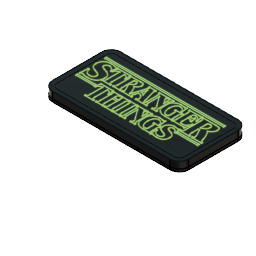
Stranger Things Lightbox (Autodesk Fusion 360 design; units mm, degrees)
part number: 2026-01-11-10-43-36-341
part number: 2026-01-17-18-05-47-932
part number: 2026-01-17-18-06-36-939
part number: 2026-01-17-18-06-53-033
Autodesk Fusion 360 part; units mm, degrees
sketch "Sketch1" plane through (0, 0, 0) normal (0, 0, 1) x (1, 0, 0)
  line L0 (-110, 55) -> (110, 55)
  line L1 (110, 55) -> (110, -55)
  line L2 (110, -55) -> (-110, -55)
  line L3 (-110, -55) -> (-110, 55)
  line L4 (-110, 55) -> (110, -55) construction
  line L5 (110, 55) -> (-110, -55) construction
  dimension "d1" = 220
  dimension "d2" = 110
  constraint horizontal L0
  constraint perpendicular L0 L1
  constraint parallel L0 L2
  constraint parallel L1 L3
  constraint coincident L4 origin
  constraint coincident L5 origin
  measures "d1" distance of L1.end L2.end
  measures "d2" distance of L0.end L1.end
extrude "Extrude1" add sketch "Sketch1" along normal blind 11 makes body 1
fillet "Fillet1" radius 15 4 edges at (110, 55, 5.5) (110, -55, 5.5) (-110, -55, 5.5) (-110, 55, 5.5) on bodies 1
shell "Shell1" thickness 7 removed faces 1 at (-31.6667, -18.3333, 0) on bodies 1
ref_plane "WorkPlane1" through (0, 0, 0) normal (0, 0, -1) x (-1, 0, 0)
sketch "Sketch4" plane through (0, 0, 0) normal (0, 0, 1) x (1, 0, 0)
  line L0 (-95, 55) -> (95, 55) construction
  line L1 (95, 48) -> (-95, 48) construction
  line L2 (0, 55) -> (0, 48) construction
  line L3 (95, 55) -> (95, 48) construction
  line L4 (0, 51.5) -> (95, 51.5) construction
  circle A0 centre (85, 51.5) radius 2.55
  line L5 (20, 0) -> (2.5, 0) construction
  circle A1 centre (85, -51.5) radius 2.55
  line L6 (0, 2.5) -> (0, 20) construction
  circle A2 centre (-85, 51.5) radius 2.55
  circle A3 centre (-85, -51.5) radius 2.55
  circle A4 centre (0, 51.5) radius 2.55
  line L7 (-103, 0) -> (-110, 0) construction
  circle A5 centre (-106.5, 0) radius 2.55
  circle A6 centre (0, -51.5) radius 2.55
  circle A7 centre (106.5, 0) radius 2.55
  point P0 (85, 51.5)
  dimension "d13" = 10
  dimension "d14" = 5.1
  dimension "d87" = 5.1
  dimension "d88" = 5.1
  constraint midpoint L0 L2.start
  constraint midpoint L1 L2.end
  constraint coincident L0.end L3.start
  constraint coincident L1.start L3.end
  constraint midpoint L2 L4.start
  constraint midpoint L3 L4.end
  constraint coincident L4 P0
  constraint coincident P0 A0.centre
  constraint symmetric A0 L5 A1
  constraint symmetric A0 L6 A2
  constraint symmetric A1 L6 A3
  constraint coincident L4.start A4.centre
  constraint horizontal L7
  constraint midpoint L7 A5.centre
  constraint symmetric L5 A4 A6
  constraint symmetric L6 A5 A7
  measures "d13" distance of L4.end P0
  measures "d14" diameter of A0
  measures "d87" diameter of A4
  measures "d88" diameter of A5
move_face "OffsetFaces1" offset -6 1 faces at (-31.6667, -16, 4) on bodies 1
extrude "Extrude4" cut sketch "Sketch4" along normal blind 3 bodies 1
sketch "Sketch5" plane through (0, 0, 0) normal (0, 0, -1) x (-1, 0, 0)
  line L0 (110, -55) -> (-110, -55)
  line L1 (-110, -55) -> (-110, 55)
  line L2 (-110, 55) -> (110, 55)
  line L3 (110, 55) -> (110, -55)
  line L4 (110, -55) -> (-110, 55) construction
  line L5 (-110, -55) -> (110, 55) construction
  dimension "d20" = 220
  dimension "d21" = 110
  constraint horizontal L0
  constraint perpendicular L0 L1
  constraint parallel L0 L2
  constraint parallel L1 L3
  constraint coincident L4 origin
  constraint coincident L5 origin
  measures "d20" distance of L1.end L2.end
  measures "d21" distance of L0.end L1.end
extrude "Extrude6" add sketch "Sketch5" along normal blind 4 separate body makes body 2
fillet "Fillet2" radius 15 4 edges at (110, 55, -2) (110, -55, -2) (-110, -55, -2) (-110, 55, -2) on bodies 2
extrude "Extrude7" cut sketch "Sketch4" against normal blind 3 bodies 2
sketch "Sketch6" plane through (0, 0, -4) normal (0, 0, -1) x (1, 0, 0)
  arc A0 (-110, -40) -> (-95, -55) centre (-95, -40) ccw
  line L0 (-95, -55) -> (95, -55)
  arc A1 (95, -55) -> (110, -40) centre (95, -40) ccw
  line L1 (110, -40) -> (110, 40)
  arc A2 (110, 40) -> (95, 55) centre (95, 40) ccw
  line L2 (95, 55) -> (-95, 55)
  arc A3 (-95, 55) -> (-110, 40) centre (-95, 40) ccw
  line L3 (-110, 40) -> (-110, -40)
  circle A4 centre (0, 40) radius 4.25
  dimension "d28" = 15
  dimension "d53" = 8.5
  measures "d28" distance of L2 A4.centre
  measures "d53" diameter of A4
sketch "Sketch7" plane through (0, 0, -4) normal (0, 0, -1) x (1, 0, 0)
  arc A0 (-110, -40) -> (-95, -55) centre (-95, -40) ccw
  line L0 (-95, -55) -> (95, -55)
  arc A1 (95, -55) -> (110, -40) centre (95, -40) ccw
  line L1 (110, -40) -> (110, 40)
  arc A2 (110, 40) -> (95, 55) centre (95, 40) ccw
  line L2 (95, 55) -> (-95, 55)
  arc A3 (-95, 55) -> (-110, 40) centre (-95, 40) ccw
  line L3 (-110, 40) -> (-110, -40)
  line L4 (0, 55) -> (95, 55) construction
  line L5 (47.5, 55) -> (57.5, 55)
  line L6 (57.5, 55) -> (57.5, 30.0008)
  line L7 (57.5, 30.0008) -> (37.5, 30.0008)
  line L8 (37.5, 30.0008) -> (37.8912, 55)
  line L9 (0, -2.5) -> (0, -20)
  line L10 (-57.5, 30.0008) -> (-37.5, 30.0008)
  line L11 (-57.5, 55) -> (-57.5, 30.0008)
  line L12 (-37.5, 30.0008) -> (-37.8912, 55)
  point P0 (47.5, 55)
  dimension "d31" = 10
  dimension "d32" = 20
  constraint midpoint L2 L4.start
  constraint coincident A2.end L2.start
  constraint midpoint L4 P0
  constraint coincident P0 L5.start
  constraint parallel L2 L5
  constraint perpendicular L5 L6
  constraint perpendicular L6 L7
  constraint coincident L2 L8.end
  constraint symmetric L5.end L9 L11.start
  constraint symmetric L6.end L9 L10.start
  constraint symmetric L7.end L9 L10.end
  constraint symmetric L8.end L9 L12.end
  measures "d31" distance of P0 L5.end
  measures "d32" distance of L6.end L7.end
extrude "Extrude9" add sketch "Sketch7" along normal blind 20 separate body contours L2 L10 L11 L12 | L2 L5 L6 L7 L8 makes body 3 at (-37.6304, -38.3339, -10.6667) makes body 4 at (37.6304, -38.3339, -17.3333)
sketch "Sketch8" plane through (57.5, 0, 0) normal (1, 0, 0) x (0, 1, 0)
  line L0 (-55, -4) -> (-55, -24)
  line L1 (-55, -24) -> (-30.0008, -24)
  line L2 (-30.0008, -24) -> (-30.0008, -4)
  circle A0 centre (-30.0008, -24) radius 18.75
  line L3 (-30.0008, -4) -> (-55, -4)
  dimension "d35" = 37.5
  constraint coincident L1.end L2.start
  measures "d35" diameter of A0
extrude "Extrude10" cut sketch "Sketch8" against normal blind 120 contours L1 L2 A0 picked at (-42.4372, -23.1105) bodies 4 2 3
fillet "Fillet3" radius 10 4 edges at (-47.5, -30.0008, -5.25) (-47.6467, -48.7508, -24) (47.6467, -48.7508, -24) (47.5, -30.0008, -5.25) on bodies 3 4
sketch "Sketch9" plane through (0, 0, 0) normal (0, 0, 1) x (-1, 0, 0)
  arc A0 (95, -55) -> (110, -40) centre (95, -40) ccw
  line L0 (110, -40) -> (110, 40)
  arc A1 (110, 40) -> (95, 55) centre (95, 40) ccw
  line L1 (95, 55) -> (-95, 55)
  arc A2 (-95, 55) -> (-110, 40) centre (-95, 40) ccw
  line L2 (-110, 40) -> (-110, -40)
  arc A3 (-110, -40) -> (-95, -55) centre (-95, -40) ccw
  line L3 (-95, -55) -> (95, -55)
  circle A4 centre (-85, -51.5) radius 2.55
  circle A5 centre (85, -51.5) radius 2.55
  circle A6 centre (-85, 51.5) radius 2.55
  circle A7 centre (85, 51.5) radius 2.55
  line L4 (102.8, -40) -> (102.8, 40)
  arc A8 (102.8, 40) -> (95, 47.8) centre (95, 40) ccw
  line L5 (95, 47.8) -> (-95, 47.8)
  arc A9 (-95, 47.8) -> (-102.8, 40) centre (-95, 40) ccw
  line L6 (-102.8, 40) -> (-102.8, -40)
  arc A10 (-102.8, -40) -> (-95, -47.8) centre (-95, -40) ccw
  line L7 (-95, -47.8) -> (95, -47.8)
  arc A11 (95, -47.8) -> (102.8, -40) centre (95, -40) ccw
  line L8 (101.6, -40) -> (101.6, 40)
  arc A12 (101.6, 40) -> (95, 46.6) centre (95, 40) ccw
  line L9 (95, 46.6) -> (-95, 46.6)
  arc A13 (-95, 46.6) -> (-101.6, 40) centre (-95, 40) ccw
  line L10 (-101.6, 40) -> (-101.6, -40)
  arc A14 (-101.6, -40) -> (-95, -46.6) centre (-95, -40) ccw
  line L11 (-95, -46.6) -> (95, -46.6)
  arc A15 (95, -46.6) -> (101.6, -40) centre (95, -40) ccw
  circle A16 centre (-106.5, 0) radius 2.55
  circle A17 centre (0, 51.5) radius 2.55
  circle A18 centre (106.5, 0) radius 2.55
  circle A19 centre (0, -51.5) radius 2.55
  dimension "d40" = -7.2
  dimension "d45" = -1.2
extrude "Extrude11" cut sketch "Sketch9" against normal blind 4 contours L4 A8 L5 A9 L6 A10 L7 A11 | L8 A12 L9 A13 L10 A14 L11 A15 bodies 3 4 2
extrude "Extrude12" add sketch "Sketch9" against normal blind 4 separate body contours L4 A8 L5 A9 L6 A10 L7 A11 | L8 A12 L9 A13 L10 A14 L11 A15 makes body 5
extrude "Extrude13" add sketch "Sketch9" along normal blind 9.5 contours L4 A8 L5 A9 L6 A10 L7 A11 bodies 3 4 2 5
sketch "Sketch10" plane through (0, -55, 0) normal (0, -1, 0) x (1, 0, 0)
  line L0 (57.5, -4) -> (37.8912, -4)
  line L1 (37.8912, -4) -> (37.8912, -24)
  line L2 (57.5, -24) -> (57.5, -4)
  line L3 (47.6956, -4) -> (47.6956, -24) construction
  line L4 (-95, 0) -> (95, 0) construction
  line L5 (57.5, -4) -> (57.5, 0) construction
  line L6 (57.5, -2) -> (31, -2) construction
  line L7 (55, -4) -> (56.1547, -2)
  line L8 (55, -4) -> (57.3094, -4) construction
  line L9 (56.1547, -2) -> (51.1547, -2)
  line L10 (51.1547, -2) -> (52.3094, -4)
  line L11 (51.1547, -2) -> (53.4641, -2) construction
  line L12 (54.9134, -3.95) -> (55.9815, -2.1)
  line L13 (55.9815, -2.1) -> (51.3279, -2.1)
  line L14 (51.3279, -2.1) -> (52.396, -3.95)
  line L15 (47.6956, -4) -> (47.6956, -2) construction
  line L16 (39.4098, -2.1) -> (44.0633, -2.1)
  line L17 (44.0633, -2.1) -> (42.9952, -3.95)
  line L18 (40.4779, -3.95) -> (39.4098, -2.1)
  line L19 (39.2365, -2) -> (44.2365, -2)
  line L20 (44.2365, -2) -> (43.0818, -4)
  line L21 (40.3912, -4) -> (39.2365, -2)
  line L22 (54.9134, -3.95) -> (54.8845, -4)
  line L23 (54.9134, -3.95) -> (54.9505, -3.95) construction
  line L24 (52.396, -3.95) -> (52.4249, -4)
  line L25 (52.396, -3.95) -> (52.5994, -3.95) construction
  line L26 (42.9952, -3.95) -> (42.9664, -4)
  line L27 (40.4779, -3.95) -> (40.5067, -4)
  line L28 (95, -4) -> (-95, -4)
  line L29 (0, -4) -> (0, 0) construction
  line L30 (-55, -4) -> (-56.1547, -2)
  line L31 (-51.1547, -2) -> (-52.3094, -4)
  line L32 (-56.1547, -2) -> (-51.1547, -2)
  line L33 (-54.9134, -3.95) -> (-54.8845, -4)
  line L34 (-55.9815, -2.1) -> (-51.3279, -2.1)
  line L35 (-51.3279, -2.1) -> (-52.396, -3.95)
  line L36 (-52.396, -3.95) -> (-52.4249, -4)
  line L37 (-54.9134, -3.95) -> (-55.9815, -2.1)
  line L38 (-40.3912, -4) -> (-39.2365, -2)
  line L39 (-39.2365, -2) -> (-44.2365, -2)
  line L40 (-44.2365, -2) -> (-43.0818, -4)
  line L41 (-40.4779, -3.95) -> (-39.4098, -2.1)
  line L42 (-39.4098, -2.1) -> (-44.0633, -2.1)
  line L43 (-44.0633, -2.1) -> (-42.9952, -3.95)
  line L44 (-42.9952, -3.95) -> (-42.9664, -4)
  line L45 (-40.4779, -3.95) -> (-40.5067, -4)
  line L46 (37.8912, -24) -> (57.5, -24)
  point P0 (55, -4)
  point P1 (47.6956, -4)
  point P2 (40.3912, -4)
  point P3 (57.5, -2)
  dimension "d56" = 2.5
  dimension "d57" = 60
  dimension "d58" = 5
  dimension "d59" = 60
  dimension "d60" = -0.1
  dimension "d61" = 120
  dimension "d62" = 60
  constraint coincident L0 P0
  constraint midpoint L0 P1
  constraint coincident P1 L3.start
  constraint symmetric P0 L3 P2
  constraint coincident L0.start L2.end
  constraint coincident L4 L5.end
  constraint perpendicular L0 L5
  constraint midpoint L5 P3
  constraint coincident P3 L6.start
  constraint perpendicular L5 L6
  constraint horizontal L8
  constraint coincident P0 L7.start
  constraint coincident L6 L7.end
  constraint parallel L6 L9
  constraint horizontal L11
  constraint coincident L0 L10.end
  constraint coincident L6 L15.end
  constraint perpendicular L6 L15
  constraint symmetric P0 L15 P2
  constraint symmetric L7.end L15 L19.start
  constraint symmetric L9.end L15 L19.end
  constraint symmetric L10.end L15 L20.end
  constraint symmetric L12.start L15 L18.start
  constraint symmetric L12.end L15 L16.start
  constraint symmetric L13.end L15 L16.end
  constraint symmetric L14.end L15 L17.end
  constraint horizontal L23
  constraint coincident L0 L22.end
  constraint horizontal L25
  constraint coincident L0 L24.end
  constraint symmetric L15 L22.end L27.end
  constraint symmetric L15 L24.end L26.end
  constraint midpoint L28 L29.start
  constraint coincident L29.end origin
  constraint symmetric P0 L29 L30.start
  constraint symmetric L7.end L29 L30.end
  constraint symmetric L9.end L29 L31.start
  constraint symmetric L10.end L29 L31.end
  constraint symmetric L12.start L29 L33.start
  constraint symmetric L12.end L29 L34.start
  constraint symmetric L13.end L29 L34.end
  constraint symmetric L14.end L29 L35.end
  constraint symmetric L16.start L29 L41.end
  constraint symmetric L16.end L29 L42.end
  constraint symmetric L17.end L29 L43.end
  constraint symmetric L18.start L29 L41.start
  constraint symmetric L19.start L29 L38.end
  constraint symmetric L19.end L29 L39.end
  constraint symmetric L20.end L29 L40.end
  constraint symmetric P2 L29 L38.start
  constraint symmetric L22.end L29 L33.end
  constraint symmetric L24.end L29 L36.end
  constraint symmetric L26.end L29 L44.end
  constraint symmetric L27.end L29 L45.end
  measures "d56" distance of L0.start P0
  measures "d57" angle of L7 L8
  measures "d58" distance of L7.end L9.end
  measures "d59" angle of L10 L11
  measures "d61" angle of L22 L23
  measures "d62" angle of L24 L25
extrude "Extrude16" cut sketch "Sketch6" against normal blind 5 contours A4 bodies 2
extrude "Extrude17" cut sketch "Sketch10" against normal blind 60 contours L0 L7 L9 L10 L12 L13 L14 L22 L24 L28 | L0 L12 L13 L14 L22 L24 L28 | L0 L16 L17 L18 L19 L20 L21 L26 L27 L28 | L0 L16 L17 L18 L26 L27 L28 | L28 L38 L39 L40 L41 L42 L43 L44 L45 | L28 L41 L42 L43 L44 L45 | L28 L30 L31 L32 L33 L34 L35 L36 L37 | L28 L33 L34 L35 L36 L37 bodies 2
extrude "Extrude18" add sketch "Sketch10" against normal blind 24 contours L0 L12 L13 L14 L22 L24 L28 | L0 L16 L17 L18 L26 L27 L28 | L28 L41 L42 L43 L44 L45 | L28 L33 L34 L35 L36 L37 bodies 3 4
sketch "Sketch11" plane through (0, 0, -4) normal (0, 0, -1) x (1, 0, 0)
  line L0 (37.5, 30.0008) -> (57.5, 30.0008)
  line L1 (57.5, 30.0008) -> (57.5, -4.9992)
  line L2 (57.5, -4.9992) -> (37.5, -4.9992)
  line L3 (37.5, -4.9992) -> (37.5, 30.0008)
  line L4 (40.3912, 55) -> (-40.3912, 55) construction
  line L5 (-95, -55) -> (95, -55) construction
  line L6 (0, 55) -> (0, -55) construction
  line L7 (-57.5, 30.0008) -> (-57.5, -4.9992)
  line L8 (-57.5, -4.9992) -> (-37.5, -4.9992)
  line L9 (-37.5, 30.0008) -> (-57.5, 30.0008)
  line L10 (-37.5, -4.9992) -> (-37.5, 30.0008)
  point P0 (37.5, 30.0008)
  dimension "d67" = 20
  dimension "d68" = 35
  constraint horizontal L0
  constraint vertical L1
  constraint horizontal L2
  constraint vertical L3
  constraint coincident P0 L0.start
  constraint midpoint L4 L6.start
  constraint midpoint L5 L6.end
  constraint symmetric P0 L6 L9.start
  constraint symmetric L0.end L6 L7.start
  constraint symmetric L1.end L6 L7.end
  constraint symmetric L2.end L6 L8.end
  measures "d67" distance of P0 L0.end
  measures "d68" distance of P0 L2.end
extrude "Extrude19" cut sketch "Sketch11" against normal blind 2 bodies 2 4
extrude "Extrude20" cut sketch "Sketch10" against normal blind 1.4 contours L0 L7 L9 L10 L12 L13 L14 L22 L24 L28 | L0 L12 L13 L14 L22 L24 L28 | L0 L16 L17 L18 L19 L20 L21 L26 L27 L28 | L0 L16 L17 L18 L26 L27 L28 bodies 4
sketch "Sketch12" plane through (0, -55, 0) normal (0, -1, 0) x (1, 0, 0)
  line L0 (-37.8912, -4) -> (-40.5067, -4)
  line L1 (-40.5067, -4) -> (-39.4098, -2.1)
  line L2 (-39.4098, -2.1) -> (-44.0633, -2.1)
  line L3 (-44.0633, -2.1) -> (-42.9664, -4)
  line L4 (-42.9664, -4) -> (-52.4249, -4)
  line L5 (-52.4249, -4) -> (-51.3279, -2.1)
  line L6 (-51.3279, -2.1) -> (-55.9815, -2.1)
  line L7 (-55.9815, -2.1) -> (-54.8845, -4)
  line L8 (-54.8845, -4) -> (-57.5, -4)
  line L9 (-57.5, -4) -> (-57.5, -24)
  line L10 (-37.8912, -24) -> (-37.8912, -4)
  line L11 (-57.5, -24) -> (-37.8912, -24)
extrude "Extrude24" cut sketch "Sketch10" against normal blind 1.4 contours L28 L41 L42 L43 L44 L45 | L28 L33 L34 L35 L36 L37 bodies 3
extrude "Extrude25" add sketch "Sketch10" against normal blind 1 contours L0 L7 L9 L10 L12 L13 L14 L22 L24 L28 | L0 L12 L13 L14 L22 L24 L28 | L0 L16 L17 L18 L19 L20 L21 L26 L27 L28 | L0 L16 L17 L18 L26 L27 L28 | L28 L38 L39 L40 L41 L42 L43 L44 L45 | L28 L41 L42 L43 L44 L45 | L28 L30 L31 L32 L33 L34 L35 L36 L37 | L28 L33 L34 L35 L36 L37 bodies 2
move_body "Move1" bodies 4 to x (1, 0, 0) y (0, 1, 0) z (0, 0, 1) at (0, -48, 0)
move_body "Move2" bodies 3 to x (1, 0, 0) y (0, 1, 0) z (0, 0, 1) at (0, -56, 0)
copy_body "Body->Comp1" bodies 1 removing the originals makes body 6 in component "Front"
copy_body "CutPasteBodies1" [suppressed] in component "Front"
copy_body "Body->Comp2" bodies 2 removing the originals makes body 7 in component "back"
copy_body "Body->Comp3" bodies 3 removing the originals makes body 8 in component "feet"
copy_body "CutPasteBodies1'" bodies 4 removing the originals makes body 9 in component "feet"
sketch "Sketch14" plane through (0, 0, 11) normal (0, 0, 1) x (-1, 0, 0)
  arc A0 (95, -55) -> (110, -40) centre (95, -40) ccw
  line L0 (110, -40) -> (110, 40)
  arc A1 (110, 40) -> (95, 55) centre (95, 40) ccw
  line L1 (95, 55) -> (-95, 55)
  arc A2 (-95, 55) -> (-110, 40) centre (-95, 40) ccw
  line L2 (-110, 40) -> (-110, -40)
  arc A3 (-110, -40) -> (-95, -55) centre (-95, -40) ccw
  line L3 (-95, -55) -> (95, -55)
  line L4 (-63.9921, 11.0113) -> (-63.9921, 13.5797)
  line L5 (-63.9921, 13.5797) -> (-97.9478, 13.5797)
  line L6 (-97.9478, 13.5797) -> (-97.9478, 11.0113)
  line L7 (-97.9478, 11.0113) -> (-63.9921, 11.0113)
  line L8 (98.4165, 11.0113) -> (98.4165, 13.5797)
  line L9 (98.4165, 13.5797) -> (69.3339, 13.5797)
  line L10 (69.3339, 13.5797) -> (69.3339, 11.0113)
  line L11 (69.3339, 11.0113) -> (98.4165, 11.0113)
  line L12 (5.43, 6.5808) -> (5.43, 7.6535)
  spline S0 degree 3 poles (5.43, 7.6535) (3.9576, 7.6106) (3.4548, 8.9411) (3.4548, 11.9451) knots 0 0 0 0 1 1 1 1
  line L13 (3.4548, 11.9451) -> (3.4548, 29.4542)
  spline S1 degree 3 poles (3.4548, 29.4542) (3.4548, 32.4581) (3.9576, 33.7883) (5.43, 33.7454) knots 0 0 0 0 1 1 1 1
  line L14 (5.43, 33.7454) -> (5.43, 34.8181)
  line L15 (5.43, 34.8181) -> (-1.5367, 34.8181)
  line L16 (-1.5367, 34.8181) -> (-1.5367, 33.7454)
  spline S2 degree 3 poles (-1.5367, 33.7454) (-0.0644, 33.7883) (0.4023, 32.4581) (0.4023, 29.4542) knots 0 0 0 0 1 1 1 1
  line L17 (0.4023, 29.4542) -> (0.4023, 11.6874)
  line L18 (0.4023, 11.6874) -> (-10.2631, 26.3641)
  spline S3 degree 3 poles (-10.2631, 26.3641) (-11.3404, 27.8232) (-12.3817, 29.2394) (-12.3817, 31.2993) knots 0 0 0 0 1 1 1 1
  spline S4 degree 3 poles (-12.3817, 31.2993) (-12.3817, 32.7584) (-11.6995, 33.5308) (-10.5503, 33.7454) knots 0 0 0 0 1 1 1 1
  line L19 (-10.5503, 33.7454) -> (-10.5503, 34.7752)
  line L20 (-10.5503, 34.7752) -> (-17.7686, 34.7752)
  line L21 (-17.7686, 34.7752) -> (-17.7686, 33.7024)
  spline S5 degree 3 poles (-17.7686, 33.7024) (-16.2963, 33.7454) (-15.7935, 32.4152) (-15.7935, 29.4112) knots 0 0 0 0 1 1 1 1
  line L22 (-15.7935, 29.4112) -> (-15.7935, 11.9451)
  spline S6 degree 3 poles (-15.7935, 11.9451) (-15.7935, 8.9411) (-16.2963, 7.6106) (-17.7686, 7.6535) knots 0 0 0 0 1 1 1 1
  line L23 (-17.7686, 7.6535) -> (-17.7686, 6.5808)
  line L24 (-17.7686, 6.5808) -> (-10.5503, 6.5808)
  line L25 (-10.5503, 6.5808) -> (-10.5503, 7.6535)
  spline S7 degree 3 poles (-10.5503, 7.6535) (-12.0227, 7.6106) (-12.741, 8.9411) (-12.741, 11.9451) knots 0 0 0 0 1 1 1 1
  line L26 (-12.741, 11.9451) -> (-12.741, 17.3521)
  line L27 (-12.741, 17.3521) -> (-8.7907, 11.5589)
  spline S8 degree 3 poles (-8.7907, 11.5589) (-8.3239, 10.9152) (-7.3544, 9.7137) (-7.3544, 8.8125) knots 0 0 0 0 1 1 1 1
  spline S9 degree 3 poles (-7.3544, 8.8125) (-7.3544, 8.1259) (-7.7852, 7.8252) (-8.2879, 7.6535) knots 0 0 0 0 1 1 1 1
  line L28 (-8.2879, 7.6535) -> (-8.2879, 6.5808)
  line L29 (-8.2879, 6.5808) -> (5.43, 6.5808)
  line L30 (17.9102, 6.5808) -> (17.9102, 7.6535)
  spline S10 degree 3 poles (17.9102, 7.6535) (16.4379, 7.6106) (15.9351, 8.9411) (15.9351, 11.9451) knots 0 0 0 0 1 1 1 1
  line L31 (15.9351, 11.9451) -> (15.9351, 29.4542)
  spline S11 degree 3 poles (15.9351, 29.4542) (15.9351, 32.4581) (16.4379, 33.7883) (17.9102, 33.7454) knots 0 0 0 0 1 1 1 1
  line L32 (17.9102, 33.7454) -> (17.9102, 34.8181)
  line L33 (17.9102, 34.8181) -> (6.5982, 34.8181)
  line L34 (6.5982, 34.8181) -> (6.5982, 33.7454)
  spline S12 degree 3 poles (6.5982, 33.7454) (8.0705, 33.7883) (8.5733, 32.4581) (8.5733, 29.4542) knots 0 0 0 0 1 1 1 1
  line L35 (8.5733, 29.4542) -> (8.5733, 11.9451)
  spline S13 degree 3 poles (8.5733, 11.9451) (8.5733, 8.9411) (8.0705, 7.6106) (6.5982, 7.6535) knots 0 0 0 0 1 1 1 1
  line L36 (6.5982, 7.6535) -> (6.5982, 6.5808)
  line L37 (6.5982, 6.5808) -> (17.9102, 6.5808)
  line L38 (45.3364, 6.5808) -> (45.3364, 7.6535)
  spline S14 degree 3 poles (45.3364, 7.6535) (43.8641, 7.6106) (43.3613, 8.9411) (43.3613, 11.9451) knots 0 0 0 0 1 1 1 1
  line L39 (43.3613, 11.9451) -> (43.3613, 29.4542)
  spline S15 degree 3 poles (43.3613, 29.4542) (43.3613, 32.4581) (43.8641, 33.7883) (45.3364, 33.7454) knots 0 0 0 0 1 1 1 1
  line L40 (45.3364, 33.7454) -> (45.3364, 34.8181)
  line L41 (45.3364, 34.8181) -> (33.8809, 34.8181)
  line L42 (33.8809, 34.8181) -> (33.8809, 33.7454)
  spline S16 degree 3 poles (33.8809, 33.7454) (35.4969, 33.7025) (35.9995, 32.415) (35.9995, 29.2394) knots 0 0 0 0 1 1 1 1
  line L43 (35.9995, 29.2394) -> (35.9995, 17.0947)
  line L44 (35.9995, 17.0947) -> (28.8533, 17.0947)
  line L45 (28.8533, 17.0947) -> (28.8533, 29.2394)
  spline S17 degree 3 poles (28.8533, 29.2394) (28.8533, 32.415) (29.3559, 33.7025) (30.9719, 33.7454) knots 0 0 0 0 1 1 1 1
  line L46 (30.9719, 33.7454) -> (30.9719, 34.8181)
  line L47 (30.9719, 34.8181) -> (19.5164, 34.8181)
  line L48 (19.5164, 34.8181) -> (19.5164, 33.7454)
  spline S18 degree 3 poles (19.5164, 33.7454) (20.9888, 33.7883) (21.4916, 32.4581) (21.4916, 29.4542) knots 0 0 0 0 1 1 1 1
  line L49 (21.4916, 29.4542) -> (21.4916, 11.9451)
  spline S19 degree 3 poles (21.4916, 11.9451) (21.4916, 8.9411) (20.9888, 7.6106) (19.5164, 7.6535) knots 0 0 0 0 1 1 1 1
  line L50 (19.5164, 7.6535) -> (19.5164, 6.5808)
  line L51 (19.5164, 6.5808) -> (30.9719, 6.5808)
  line L52 (30.9719, 6.5808) -> (30.9719, 7.6535)
  spline S20 degree 3 poles (30.9719, 7.6535) (29.4995, 7.6106) (28.8533, 8.9411) (28.8533, 11.9451) knots 0 0 0 0 1 1 1 1
  line L53 (28.8533, 11.9451) -> (28.8533, 14.2624)
  line L54 (28.8533, 14.2624) -> (35.9995, 14.2624)
  line L55 (35.9995, 14.2624) -> (35.9995, 11.9451)
  spline S21 degree 3 poles (35.9995, 11.9451) (35.9995, 8.9411) (35.3533, 7.6106) (33.8809, 7.6535) knots 0 0 0 0 1 1 1 1
  line L56 (33.8809, 7.6535) -> (33.8809, 6.5808)
  line L57 (33.8809, 6.5808) -> (45.3364, 6.5808)
  spline S22 degree 3 poles (-61.5928, 5.7654) (-61.09, 6.4949) (-60.0847, 6.7956) (-59.3664, 6.7956) knots 0 0 0 0 1 1 1 1
  spline S23 degree 3 poles (-59.3664, 6.7956) (-58.6123, 6.7956) (-56.4577, 5.8943) (-52.7947, 5.8943) knots 0 0 0 0 1 1 1 1
  spline S24 degree 3 poles (-52.7947, 5.8943) (-49.6705, 5.8943) (-43.7451, 7.6106) (-43.7451, 15.3351) knots 0 0 0 0 1 1 1 1
  spline S25 degree 3 poles (-43.7451, 15.3351) (-43.7451, 17.3091) (-44.5713, 19.2831) (-45.8641, 20.5276) knots 0 0 0 0 1 1 1 1
  spline S26 degree 3 poles (-45.8641, 20.5276) (-46.9773, 21.6005) (-48.6649, 22.3303) (-50.0295, 22.8453) knots 0 0 0 0 1 1 1 1
  line L58 (-50.0295, 22.8453) -> (-53.6565, 24.2612)
  spline S27 degree 3 poles (-53.6565, 24.2612) (-55.1648, 24.862) (-57.3556, 25.4631) (-57.3556, 27.8234) knots 0 0 0 0 1 1 1 1
  spline S28 degree 3 poles (-57.3556, 27.8234) (-57.3556, 31.3853) (-54.5544, 32.0717) (-52.1124, 32.0717) knots 0 0 0 0 1 1 1 1
  spline S29 degree 3 poles (-52.1124, 32.0717) (-48.3921, 32.0717) (-45.3265, 29.2409) (-44.1447, 25.2239) knots 0 0 0 0 1 1 1 1
  line L59 (-44.1447, 25.2239) -> (-43.0697, 25.2239)
  line L60 (-43.0697, 25.2239) -> (-43.7451, 35.4621)
  spline S30 degree 3 poles (-43.7451, 35.4621) (-44.2838, 34.8183) (-44.8582, 34.4319) (-45.6842, 34.4319) knots 0 0 0 0 1 1 1 1
  spline S31 degree 3 poles (-45.6842, 34.4319) (-46.3665, 34.4319) (-47.3721, 34.6894) (-48.0544, 34.8611) knots 0 0 0 0 1 1 1 1
  spline S32 degree 3 poles (-48.0544, 34.8611) (-49.8499, 35.2473) (-51.2505, 35.5046) (-53.082, 35.5046) knots 0 0 0 0 1 1 1 1
  spline S33 degree 3 poles (-53.082, 35.5046) (-60.4437, 35.5046) (-64.9686, 32.2437) (-64.9686, 25.1199) knots 0 0 0 0 1 1 1 1
  spline S34 degree 3 poles (-64.9686, 25.1199) (-64.9686, 21.5152) (-62.2754, 18.6396) (-59.0074, 17.4809) knots 0 0 0 0 1 1 1 1
  line L61 (-59.0074, 17.4809) -> (-54.8056, 15.979)
  spline S35 degree 3 poles (-54.8056, 15.979) (-53.4769, 15.507) (-51.0708, 14.8633) (-51.0708, 12.7175) knots 0 0 0 0 1 1 1 1
  spline S36 degree 3 poles (-51.0708, 12.7175) (-50.963, 10.2714) (-53.2614, 9.3272) (-55.0211, 9.3272) knots 0 0 0 0 1 1 1 1
  spline S37 degree 3 poles (-55.0211, 9.3272) (-57.413, 9.3272) (-59.8038, 11.2316) (-61.118, 13.6771) knots 0 0 0 0 1 1 1 1
  line L62 (-61.118, 13.6771) -> (-62.3859, 13.6771)
  line L63 (-62.3859, 13.6771) -> (-61.5928, 5.7654)
  line L64 (66.0076, 5.6454) -> (67.5194, 14.0495)
  line L65 (67.5194, 14.0495) -> (66.5898, 14.0495)
  spline S38 degree 3 poles (66.5898, 14.0495) (65.4852, 10.7623) (63.0759, 8.9616) (59.9441, 8.8819) knots 0 0 0 0 1 1 1 1
  line L66 (59.9441, 8.8819) -> (59.9441, 29.0545)
  spline S39 degree 3 poles (59.9441, 29.0545) (59.9441, 32.2467) (60.4634, 33.6654) (62.875, 33.7097) knots 0 0 0 0 1 1 1 1
  line L67 (62.875, 33.7097) -> (62.875, 34.8185)
  line L68 (62.875, 34.8185) -> (49.4071, 34.8185)
  line L69 (49.4071, 34.8185) -> (49.4071, 33.7097)
  spline S40 degree 3 poles (49.4071, 33.7097) (51.8187, 33.6654) (52.3384, 32.2467) (52.3384, 29.0545) knots 0 0 0 0 1 1 1 1
  line L70 (52.3384, 29.0545) -> (52.3384, 8.8819)
  spline S41 degree 3 poles (52.3384, 8.8819) (49.0823, 9.1202) (47.0782, 10.8563) (45.7886, 14.0495) knots 0 0 0 0 1 1 1 1
  line L71 (45.7886, 14.0495) -> (44.7895, 14.0495)
  line L72 (44.7895, 14.0495) -> (46.2082, 5.6454)
  line L73 (46.2082, 5.6454) -> (66.0076, 5.6454)
  spline S42 degree 3 poles (-38.2841, 5.594) (-37.8172, 6.3664) (-37.099, 6.7956) (-36.309, 6.7956) knots 0 0 0 0 1 1 1 1
  spline S43 degree 3 poles (-36.309, 6.7956) (-35.7703, 6.7956) (-35.2314, 6.667) (-34.6928, 6.5382) knots 0 0 0 0 1 1 1 1
  spline S44 degree 3 poles (-34.6928, 6.5382) (-32.8613, 6.1091) (-31.784, 5.8947) (-29.0906, 5.8947) knots 0 0 0 0 1 1 1 1
  spline S45 degree 3 poles (-29.0906, 5.8947) (-23.635, 5.8947) (-18.8455, 8.3985) (-16.8566, 13.6637) knots 0 0 0 0 1 1 1 1
  line L74 (-16.8566, 13.6637) -> (-16.8566, 25.3597)
  spline S46 degree 3 poles (-16.8566, 25.3597) (-17.6945, 27.8165) (-19.0416, 30.0345) (-20.7954, 31.6429) knots 0 0 0 0 1 1 1 1
  spline S47 degree 3 poles (-20.7954, 31.6429) (-23.8479, 34.4323) (-27.6542, 34.8185) (-31.3531, 34.8185) knots 0 0 0 0 1 1 1 1
  line L75 (-31.3531, 34.8185) -> (-42.9163, 34.8185)
  line L76 (-42.9163, 34.8185) -> (-42.9163, 33.7458)
  spline S48 degree 3 poles (-42.9163, 33.7458) (-42.3417, 33.4883) (-41.7316, 33.2308) (-41.4443, 32.5442) knots 0 0 0 0 1 1 1 1
  spline S49 degree 3 poles (-41.4443, 32.5442) (-41.0853, 31.7288) (-41.121, 29.7118) (-41.121, 28.7676) knots 0 0 0 0 1 1 1 1
  line L77 (-41.121, 28.7676) -> (-41.121, 23.7895)
  spline S50 degree 3 poles (-41.121, 23.7895) (-41.121, 21.5151) (-40.8338, 18.9834) (-43.3834, 18.8117) knots 0 0 0 0 1 1 1 1
  line L78 (-43.3834, 18.8117) -> (-43.3834, 17.739)
  line L79 (-43.3834, 17.739) -> (-31.8559, 17.739)
  line L80 (-31.8559, 17.739) -> (-31.8559, 18.8117)
  spline S51 degree 3 poles (-31.8559, 18.8117) (-34.226, 18.9405) (-34.0465, 21.215) (-34.0465, 23.3178) knots 0 0 0 0 1 1 1 1
  line L81 (-34.0465, 23.3178) -> (-34.0465, 27.2658)
  spline S52 degree 3 poles (-34.0465, 27.2658) (-34.0465, 28.2957) (-34.0825, 29.669) (-33.6515, 30.5702) knots 0 0 0 0 1 1 1 1
  spline S53 degree 3 poles (-33.6515, 30.5702) (-33.1847, 31.6001) (-32.0712, 31.9862) (-31.1375, 31.9862) knots 0 0 0 0 1 1 1 1
  spline S54 degree 3 poles (-31.1375, 31.9862) (-26.0382, 31.9862) (-23.7762, 25.0771) (-23.7762, 19.9274) knots 0 0 0 0 1 1 1 1
  spline S55 degree 3 poles (-23.7762, 19.9274) (-23.7762, 14.6061) (-25.715, 9.1132) (-30.8503, 9.1132) knots 0 0 0 0 1 1 1 1
  spline S56 degree 3 poles (-30.8503, 9.1132) (-34.3696, 9.1132) (-37.3503, 11.9453) (-38.6431, 15.7646) knots 0 0 0 0 1 1 1 1
  line L82 (-38.6431, 15.7646) -> (-39.3971, 15.6362)
  line L83 (-39.3971, 15.6362) -> (-38.2841, 5.594)
  line L84 (52.926, -28.9776) -> (52.926, -27.9045)
  spline S57 degree 3 poles (52.926, -27.9045) (51.4536, -27.9475) (50.9512, -26.6173) (50.9512, -23.6133) knots 0 0 0 0 1 1 1 1
  line L85 (50.9512, -23.6133) -> (50.9512, -6.1043)
  spline S58 degree 3 poles (50.9512, -6.1043) (50.9512, -3.1003) (51.4536, -1.7701) (52.926, -1.813) knots 0 0 0 0 1 1 1 1
  line L86 (52.926, -1.813) -> (52.926, -0.7399)
  line L87 (52.926, -0.7399) -> (41.65, -0.7399)
  line L88 (41.65, -0.7399) -> (41.65, -1.813)
  spline S59 degree 3 poles (41.65, -1.813) (43.1223, -1.7701) (43.6251, -3.1003) (43.6251, -6.1043) knots 0 0 0 0 1 1 1 1
  line L89 (43.6251, -6.1043) -> (43.6251, -13.6141)
  line L90 (43.6251, -13.6141) -> (42.3683, -14.1291)
  spline S60 degree 3 poles (42.3683, -14.1291) (40.86, -12.0263) (37.269, -5.8468) (37.269, -3.229) knots 0 0 0 0 1 1 1 1
  spline S61 degree 3 poles (37.269, -3.229) (37.269, -2.0703) (37.9154, -1.8559) (38.7413, -1.813) knots 0 0 0 0 1 1 1 1
  line L91 (38.7413, -1.813) -> (38.7413, -0.7399)
  line L92 (38.7413, -0.7399) -> (23.158, -0.7399)
  line L93 (23.158, -0.7399) -> (23.158, -1.813)
  spline S62 degree 3 poles (23.158, -1.813) (24.1276, -1.9418) (24.8098, -2.3708) (24.8098, -3.7011) knots 0 0 0 0 1 1 1 1
  spline S63 degree 3 poles (24.8098, -3.7011) (24.8098, -4.6452) (24.3789, -6.2758) (24.1275, -7.177) knots 0 0 0 0 1 1 1 1
  line L94 (24.1275, -7.177) -> (22.8347, -11.5545)
  spline S64 degree 3 poles (22.8347, -11.5545) (20.8236, -11.6833) (19.0643, -11.0393) (17.4124, -9.6661) knots 0 0 0 0 1 1 1 1
  spline S65 degree 3 poles (17.4124, -9.6661) (16.0119, -8.5503) (14.3956, -6.4049) (14.3956, -4.3021) knots 0 0 0 0 1 1 1 1
  spline S66 degree 3 poles (14.3956, -4.3021) (14.3956, -2.843) (15.2216, -1.8989) (16.3708, -1.813) knots 0 0 0 0 1 1 1 1
  line L95 (16.3708, -1.813) -> (16.3708, -0.7399)
  line L96 (16.3708, -0.7399) -> (-0.9177, -0.7399)
  line L97 (-0.9177, -0.7399) -> (-0.9177, -1.813)
  spline S67 degree 3 poles (-0.9177, -1.813) (0.5546, -1.7701) (1.0214, -3.1003) (1.0214, -6.1043) knots 0 0 0 0 1 1 1 1
  line L98 (1.0214, -6.1043) -> (1.0214, -23.8706)
  line L99 (1.0214, -23.8706) -> (-9.6441, -9.1943)
  spline S68 degree 3 poles (-9.6441, -9.1943) (-10.7214, -7.7353) (-11.763, -6.3186) (-11.763, -4.2588) knots 0 0 0 0 1 1 1 1
  spline S69 degree 3 poles (-11.763, -4.2588) (-11.763, -2.7997) (-11.0805, -2.0276) (-9.9313, -1.813) knots 0 0 0 0 1 1 1 1
  line L100 (-9.9313, -1.813) -> (-9.9313, -0.7829)
  line L101 (-9.9313, -0.7829) -> (-17.1496, -0.7829)
  line L102 (-17.1496, -0.7829) -> (-17.1496, -1.8556)
  spline S70 degree 3 poles (-17.1496, -1.8556) (-15.6773, -1.8127) (-15.1745, -3.1432) (-15.1745, -6.1472) knots 0 0 0 0 1 1 1 1
  line L103 (-15.1745, -6.1472) -> (-15.1745, -23.6133)
  spline S71 degree 3 poles (-15.1745, -23.6133) (-15.1745, -26.6173) (-15.6773, -27.9475) (-17.1496, -27.9045) knots 0 0 0 0 1 1 1 1
  line L104 (-17.1496, -27.9045) -> (-17.1496, -28.9776)
  line L105 (-17.1496, -28.9776) -> (-9.9313, -28.9776)
  line L106 (-9.9313, -28.9776) -> (-9.9313, -27.9045)
  spline S72 degree 3 poles (-9.9313, -27.9045) (-11.4037, -27.9475) (-12.122, -26.6173) (-12.122, -23.6133) knots 0 0 0 0 1 1 1 1
  line L107 (-12.122, -23.6133) -> (-12.122, -18.206)
  line L108 (-12.122, -18.206) -> (-8.1721, -23.9995)
  spline S73 degree 3 poles (-8.1721, -23.9995) (-7.7053, -24.6432) (-6.7354, -25.8447) (-6.7354, -26.7459) knots 0 0 0 0 1 1 1 1
  spline S74 degree 3 poles (-6.7354, -26.7459) (-6.7354, -27.4325) (-7.1665, -27.7329) (-7.6693, -27.9045) knots 0 0 0 0 1 1 1 1
  line L109 (-7.6693, -27.9045) -> (-7.6693, -28.9776)
  line L110 (-7.6693, -28.9776) -> (6.0486, -28.9776)
  line L111 (6.0486, -28.9776) -> (6.0486, -27.9045)
  spline S75 degree 3 poles (6.0486, -27.9045) (4.5762, -27.9475) (4.0738, -26.6173) (4.0738, -23.6133) knots 0 0 0 0 1 1 1 1
  line L112 (4.0738, -23.6133) -> (4.0738, -6.1043)
  spline S76 degree 3 poles (4.0738, -6.1043) (4.0738, -4.0603) (4.3073, -2.7928) (4.9199, -2.2038) knots 0 0 0 0 1 1 1 1
  spline S77 degree 3 poles (4.9199, -2.2038) (6.0871, -3.0854) (6.5249, -5.1992) (6.9621, -6.6623) knots 0 0 0 0 1 1 1 1
  spline S78 degree 3 poles (6.9621, -6.6623) (9.44, -15.4168) (12.5643, -26.2739) (12.5643, -26.8318) knots 0 0 0 0 1 1 1 1
  spline S79 degree 3 poles (12.5643, -26.8318) (12.5643, -27.5614) (12.2768, -27.8187) (11.7382, -27.9045) knots 0 0 0 0 1 1 1 1
  line L113 (11.7382, -27.9045) -> (11.7382, -28.9776)
  line L114 (11.7382, -28.9776) -> (22.2241, -28.9776)
  line L115 (22.2241, -28.9776) -> (22.2241, -27.9045)
  spline S80 degree 3 poles (22.2241, -27.9045) (21.7213, -27.8187) (21.4344, -27.4755) (21.4344, -26.8318) knots 0 0 0 0 1 1 1 1
  spline S81 degree 3 poles (21.4344, -26.8318) (21.4344, -26.231) (21.8651, -25.0295) (22.0446, -24.5146) knots 0 0 0 0 1 1 1 1
  line L116 (22.0446, -24.5146) -> (27.6828, -6.7053)
  spline S82 degree 3 poles (27.6828, -6.7053) (28.014, -5.7469) (28.3647, -4.6902) (28.8571, -3.7947) knots 0 0 0 0 1 1 1 1
  spline S83 degree 3 poles (28.8571, -3.7947) (29.0722, -4.3045) (29.2401, -4.8439) (29.3684, -5.3319) knots 0 0 0 0 1 1 1 1
  spline S84 degree 3 poles (29.3684, -5.3319) (30.6253, -9.9237) (32.7085, -14.2152) (35.3659, -17.2621) knots 0 0 0 0 1 1 1 1
  spline S85 degree 3 poles (35.3659, -17.2621) (32.9958, -18.7212) (30.2662, -21.0816) (30.2662, -24.6434) knots 0 0 0 0 1 1 1 1
  spline S86 degree 3 poles (30.2662, -24.6434) (30.2662, -26.36) (31.0922, -27.6041) (32.3491, -28.2908) knots 0 0 0 0 1 1 1 1
  spline S87 degree 3 poles (32.3491, -28.2908) (33.7138, -28.9345) (35.2938, -28.9347) (36.7662, -28.9776) knots 0 0 0 0 1 1 1 1
  line L117 (36.7662, -28.9776) -> (52.926, -28.9776)
  spline S88 degree 3 poles (40.896, -26.1453) (39.1004, -26.1453) (37.8795, -25.0295) (37.8795, -22.8409) knots 0 0 0 0 1 1 1 1
  spline S89 degree 3 poles (37.8795, -22.8409) (37.8795, -19.1932) (41.1832, -17.4766) (43.6251, -16.7471) knots 0 0 0 0 1 1 1 1
  line L118 (43.6251, -16.7471) -> (43.6251, -23.0982)
  spline S90 degree 3 poles (43.6251, -23.0982) (43.6251, -23.7419) (43.6968, -24.8146) (43.3018, -25.3296) knots 0 0 0 0 1 1 1 1
  spline S91 degree 3 poles (43.3018, -25.3296) (42.7631, -25.9733) (41.6142, -26.1453) (40.896, -26.1453) knots 0 0 0 0 1 1 1 1
  line L119 (19.4589, -23.27) -> (16.7297, -13.099)
  spline S92 degree 3 poles (16.7297, -13.099) (18.1662, -14.3006) (19.9257, -15.2448) (21.7213, -15.2018) knots 0 0 0 0 1 1 1 1
  line L120 (21.7213, -15.2018) -> (19.4589, -23.27)
  line L121 (-63.9921, -29.1422) -> (-63.9921, -27.7546)
  spline S93 degree 3 poles (-63.9921, -27.7546) (-65.8966, -27.8101) (-66.5468, -26.0891) (-66.5468, -22.2035) knots 0 0 0 0 1 1 1 1
  line L122 (-66.5468, -22.2035) -> (-66.5468, 0.444)
  spline S94 degree 3 poles (-66.5468, 0.444) (-66.5468, 4.3296) (-65.8966, 6.0506) (-63.9921, 5.9951) knots 0 0 0 0 1 1 1 1
  line L123 (-63.9921, 5.9951) -> (-63.9921, 7.3827)
  line L124 (-63.9921, 7.3827) -> (-78.5775, 7.3827)
  line L125 (-78.5775, 7.3827) -> (-78.5775, 5.9951)
  spline S95 degree 3 poles (-78.5775, 5.9951) (-76.6731, 6.0506) (-76.0229, 4.3296) (-76.0229, 0.444) knots 0 0 0 0 1 1 1 1
  line L126 (-76.0229, 0.444) -> (-76.0229, -9.2699)
  line L127 (-76.0229, -9.2699) -> (-77.6486, -9.9361)
  spline S96 degree 3 poles (-77.6486, -9.9361) (-79.5996, -7.2161) (-84.2445, 0.777) (-84.2445, 4.163) knots 0 0 0 0 1 1 1 1
  spline S97 degree 3 poles (-84.2445, 4.163) (-84.2445, 5.6618) (-83.4086, 5.9396) (-82.3403, 5.9951) knots 0 0 0 0 1 1 1 1
  line L128 (-82.3403, 5.9951) -> (-82.3403, 7.3827)
  line L129 (-82.3403, 7.3827) -> (-97.9478, 7.3827)
  line L130 (-97.9478, 7.3827) -> (-97.9478, 5.9951)
  spline S98 degree 3 poles (-97.9478, 5.9951) (-95.9039, 5.9951) (-94.9748, 3.3859) (-94.4639, 1.4431) knots 0 0 0 0 1 1 1 1
  spline S99 degree 3 poles (-94.4639, 1.4431) (-92.8381, -4.4964) (-90.1441, -10.0472) (-86.7067, -13.9884) knots 0 0 0 0 1 1 1 1
  spline S100 degree 3 poles (-86.7067, -13.9884) (-89.7724, -15.8757) (-93.3025, -18.9286) (-93.3025, -23.5358) knots 0 0 0 0 1 1 1 1
  spline S101 degree 3 poles (-93.3025, -23.5358) (-93.3025, -25.7562) (-92.234, -27.3658) (-90.6083, -28.2539) knots 0 0 0 0 1 1 1 1
  spline S102 degree 3 poles (-90.6083, -28.2539) (-88.8432, -29.0866) (-86.7994, -29.0867) (-84.8949, -29.1422) knots 0 0 0 0 1 1 1 1
  line L131 (-84.8949, -29.1422) -> (-63.9921, -29.1422)
  spline S103 degree 3 poles (-79.5532, -25.4788) (-81.8757, -25.4788) (-83.4548, -24.0353) (-83.4548, -21.2044) knots 0 0 0 0 1 1 1 1
  spline S104 degree 3 poles (-83.4548, -21.2044) (-83.4548, -16.4861) (-79.1815, -14.2659) (-76.0229, -13.3222) knots 0 0 0 0 1 1 1 1
  line L132 (-76.0229, -13.3222) -> (-76.0229, -21.5373)
  spline S105 degree 3 poles (-76.0229, -21.5373) (-76.0229, -22.3699) (-75.9299, -23.758) (-76.4409, -24.4241) knots 0 0 0 0 1 1 1 1
  spline S106 degree 3 poles (-76.4409, -24.4241) (-77.1377, -25.2567) (-78.6242, -25.4788) (-79.5532, -25.4788) knots 0 0 0 0 1 1 1 1
  line L133 (73.5339, -29.3662) -> (75.0373, -21.0073)
  line L134 (75.0373, -21.0073) -> (74.1126, -21.0073)
  spline S107 degree 3 poles (74.1126, -21.0073) (73.014, -24.2766) (70.6181, -26.0677) (67.5033, -26.1469) knots 0 0 0 0 1 1 1 1
  line L135 (67.5033, -26.1469) -> (67.5033, -6.0839)
  spline S108 degree 3 poles (67.5033, -6.0839) (67.5033, -2.9091) (68.0197, -1.4981) (70.4181, -1.454) knots 0 0 0 0 1 1 1 1
  line L136 (70.4181, -1.454) -> (70.4181, -0.3514)
  line L137 (70.4181, -0.3514) -> (57.0235, -0.3514)
  line L138 (57.0235, -0.3514) -> (57.0235, -1.454)
  spline S109 degree 3 poles (57.0235, -1.454) (59.422, -1.4981) (59.9387, -2.9091) (59.9387, -6.0839) knots 0 0 0 0 1 1 1 1
  line L139 (59.9387, -6.0839) -> (59.9387, -26.1469)
  spline S110 degree 3 poles (59.9387, -26.1469) (56.7003, -25.9099) (54.7071, -24.1831) (53.4245, -21.0073) knots 0 0 0 0 1 1 1 1
  line L140 (53.4245, -21.0073) -> (52.4308, -21.0073)
  line L141 (52.4308, -21.0073) -> (53.8422, -29.3662)
  line L142 (53.8422, -29.3662) -> (73.5339, -29.3662)
  spline S111 degree 3 poles (-62.0392, -29.6642) (-61.3569, -28.8059) (-59.9206, -28.9776) (-59.0228, -28.9776) knots 0 0 0 0 1 1 1 1
  line L143 (-59.0228, -28.9776) -> (-42.7192, -28.9776)
  line L144 (-42.7192, -28.9776) -> (-42.7192, -27.9045)
  spline S112 degree 3 poles (-42.7192, -27.9045) (-44.1915, -27.9475) (-44.6943, -26.6173) (-44.6943, -23.6133) knots 0 0 0 0 1 1 1 1
  line L145 (-44.6943, -23.6133) -> (-44.6943, -6.1043)
  spline S113 degree 3 poles (-44.6943, -6.1043) (-44.6943, -3.1003) (-44.1915, -1.7701) (-42.7192, -1.813) knots 0 0 0 0 1 1 1 1
  line L146 (-42.7192, -1.813) -> (-42.7192, -0.7399)
  line L147 (-42.7192, -0.7399) -> (-60.5312, -0.7399)
  spline S114 degree 3 poles (-60.5312, -0.7399) (-60.9262, -0.7399) (-61.3211, -0.7398) (-61.6802, -0.654) knots 0 0 0 0 1 1 1 1
  spline S115 degree 3 poles (-61.6802, -0.654) (-62.0752, -0.6111) (-62.3985, -0.4396) (-62.6858, -0.0534) knots 0 0 0 0 1 1 1 1
  line L148 (-62.6858, -0.0534) -> (-65.7383, -11.2109)
  line L149 (-65.7383, -11.2109) -> (-64.9843, -11.5545)
  spline S116 degree 3 poles (-64.9843, -11.5545) (-63.081, -6.8769) (-60.1359, -3.5723) (-55.5392, -3.5723) knots 0 0 0 0 1 1 1 1
  spline S117 degree 3 poles (-55.5392, -3.5723) (-52.7023, -3.5723) (-52.0561, -4.688) (-52.0561, -7.6062) knots 0 0 0 0 1 1 1 1
  line L150 (-52.0561, -7.6062) -> (-52.0561, -16.9189)
  line L151 (-52.0561, -16.9189) -> (-53.0256, -16.9189)
  spline S118 degree 3 poles (-53.0256, -16.9189) (-54.8212, -16.9189) (-56.3294, -17.0904) (-57.7299, -15.5455) knots 0 0 0 0 1 1 1 1
  spline S119 degree 3 poles (-57.7299, -15.5455) (-57.9927, -15.2599) (-58.2314, -14.9452) (-58.4479, -14.6089) knots 0 0 0 0 1 1 1 1
  line L152 (-58.4479, -14.6089) -> (-59.8711, -14.7788)
  line L153 (-59.8711, -14.7788) -> (-58.798, -22.1812)
  line L154 (-58.798, -22.1812) -> (-57.8396, -22.1812)
  spline S120 degree 3 poles (-57.8396, -22.1812) (-57.4451, -19.5194) (-55.328, -19.7508) (-53.2055, -19.7508) knots 0 0 0 0 1 1 1 1
  line L155 (-53.2055, -19.7508) -> (-52.0561, -19.7508)
  line L156 (-52.0561, -19.7508) -> (-52.0561, -21.1242)
  spline S121 degree 3 poles (-52.0561, -21.1242) (-52.0561, -24.5574) (-51.8408, -26.1453) (-55.3601, -26.1453) knots 0 0 0 0 1 1 1 1
  spline S122 degree 3 poles (-55.3601, -26.1453) (-58.9512, -26.1453) (-62.0394, -23.6561) (-63.0808, -19.4935) knots 0 0 0 0 1 1 1 1
  line L157 (-63.0808, -19.4935) -> (-63.8709, -19.7942)
  line L158 (-63.8709, -19.7942) -> (-62.0392, -29.6642)
  spline S123 degree 3 poles (-37.6647, -29.9645) (-37.1979, -29.192) (-36.48, -28.7629) (-35.6899, -28.7629) knots 0 0 0 0 1 1 1 1
  spline S124 degree 3 poles (-35.6899, -28.7629) (-35.1513, -28.7629) (-34.6124, -28.8915) (-34.0738, -29.0202) knots 0 0 0 0 1 1 1 1
  spline S125 degree 3 poles (-34.0738, -29.0202) (-32.2423, -29.4494) (-31.165, -29.6642) (-28.4716, -29.6642) knots 0 0 0 0 1 1 1 1
  spline S126 degree 3 poles (-28.4716, -29.6642) (-23.0159, -29.6642) (-18.2265, -27.1599) (-16.2376, -21.8947) knots 0 0 0 0 1 1 1 1
  line L159 (-16.2376, -21.8947) -> (-16.2376, -10.1988)
  spline S127 degree 3 poles (-16.2376, -10.1988) (-17.0755, -7.7419) (-18.4226, -5.5239) (-20.1764, -3.9155) knots 0 0 0 0 1 1 1 1
  spline S128 degree 3 poles (-20.1764, -3.9155) (-23.2289, -1.1261) (-27.0352, -0.7399) (-30.734, -0.7399) knots 0 0 0 0 1 1 1 1
  line L160 (-30.734, -0.7399) -> (-42.2973, -0.7399)
  line L161 (-42.2973, -0.7399) -> (-42.2973, -1.813)
  spline S129 degree 3 poles (-42.2973, -1.813) (-41.7227, -2.0705) (-41.1122, -2.3276) (-40.8249, -3.0142) knots 0 0 0 0 1 1 1 1
  spline S130 degree 3 poles (-40.8249, -3.0142) (-40.4658, -3.8296) (-40.502, -5.8467) (-40.502, -6.7908) knots 0 0 0 0 1 1 1 1
  line L162 (-40.502, -6.7908) -> (-40.502, -11.7689)
  spline S131 degree 3 poles (-40.502, -11.7689) (-40.502, -14.0434) (-40.2148, -16.5754) (-42.7644, -16.7471) knots 0 0 0 0 1 1 1 1
  line L163 (-42.7644, -16.7471) -> (-42.7644, -17.8198)
  line L164 (-42.7644, -17.8198) -> (-31.2368, -17.8198)
  line L165 (-31.2368, -17.8198) -> (-31.2368, -16.7471)
  spline S132 degree 3 poles (-31.2368, -16.7471) (-33.607, -16.6183) (-33.4275, -14.3438) (-33.4275, -12.241) knots 0 0 0 0 1 1 1 1
  line L166 (-33.4275, -12.241) -> (-33.4275, -8.293)
  spline S133 degree 3 poles (-33.4275, -8.293) (-33.4275, -7.2631) (-33.4631, -5.8894) (-33.0321, -4.9882) knots 0 0 0 0 1 1 1 1
  spline S134 degree 3 poles (-33.0321, -4.9882) (-32.5653, -3.9583) (-31.4522, -3.5723) (-30.5185, -3.5723) knots 0 0 0 0 1 1 1 1
  spline S135 degree 3 poles (-30.5185, -3.5723) (-25.4191, -3.5723) (-23.1568, -10.4817) (-23.1568, -15.6314) knots 0 0 0 0 1 1 1 1
  spline S136 degree 3 poles (-23.1568, -15.6314) (-23.1568, -20.9527) (-25.096, -26.4456) (-30.2312, -26.4456) knots 0 0 0 0 1 1 1 1
  spline S137 degree 3 poles (-30.2312, -26.4456) (-33.7505, -26.4456) (-36.7309, -23.6135) (-38.0237, -19.7942) knots 0 0 0 0 1 1 1 1
  line L167 (-38.0237, -19.7942) -> (-38.7781, -19.9223)
  line L168 (-38.7781, -19.9223) -> (-37.6647, -29.9645)
  spline S138 degree 3 poles (86.8042, -30.7346) (90.8396, -30.7346) (98.4122, -28.5989) (98.4165, -18.8357) knots 0 0 0 0 1 1 1 1
  spline S139 degree 3 poles (98.4165, -18.8357) (98.4191, -12.9601) (95.2348, -10.5636) (90.4204, -8.7314) knots 0 0 0 0 1 1 1 1
  line L169 (90.4204, -8.7314) -> (85.7357, -6.9024)
  spline S140 degree 3 poles (85.7357, -6.9024) (83.7875, -6.1264) (80.9577, -5.3906) (80.9577, -2.3419) knots 0 0 0 0 1 1 1 1
  spline S141 degree 3 poles (80.9577, -2.3419) (80.9577, 2.2588) (84.4546, 3.0853) (87.6088, 3.0853) knots 0 0 0 0 1 1 1 1
  spline S142 degree 3 poles (87.6088, 3.0853) (92.2612, 3.0853) (94.6563, -0.5923) (96.1533, -5.2134) knots 0 0 0 0 1 1 1 1
  line L170 (96.1533, -5.2134) -> (97.7193, -5.2134)
  line L171 (97.7193, -5.2134) -> (98.4165, 7.525)
  spline S143 degree 3 poles (98.4165, 7.525) (97.7208, 6.6936) (96.9786, 6.2556) (95.9117, 6.2556) knots 0 0 0 0 1 1 1 1
  spline S144 degree 3 poles (95.9117, 6.2556) (95.0304, 6.2556) (93.7317, 6.5876) (92.8504, 6.8094) knots 0 0 0 0 1 1 1 1
  spline S145 degree 3 poles (92.8504, 6.8094) (90.5312, 7.3082) (88.7222, 7.6408) (86.3566, 7.6408) knots 0 0 0 0 1 1 1 1
  spline S146 degree 3 poles (86.3566, 7.6408) (76.8477, 7.6408) (71.003, 3.3679) (71.003, -5.8335) knots 0 0 0 0 1 1 1 1
  spline S147 degree 3 poles (71.003, -5.8335) (71.003, -10.4896) (74.4816, -14.2038) (78.7026, -15.7004) knots 0 0 0 0 1 1 1 1
  line L172 (78.7026, -15.7004) -> (84.1302, -17.6403)
  spline S148 degree 3 poles (84.1302, -17.6403) (85.8465, -18.25) (88.8892, -19.0826) (88.9542, -21.8533) knots 0 0 0 0 1 1 1 1
  spline S149 degree 3 poles (88.9542, -21.8533) (89.0284, -25.015) (86.1247, -26.232) (83.8518, -26.232) knots 0 0 0 0 1 1 1 1
  spline S150 degree 3 poles (83.8518, -26.232) (80.7623, -26.232) (77.6134, -23.5098) (75.9159, -20.351) knots 0 0 0 0 1 1 1 1
  line L173 (75.9159, -20.351) -> (74.2932, -29.3746)
  spline S151 degree 2 poles (74.2932, -29.3746) (74.8052, -28.9767) (76.2227, -29.1679) knots 0 0 0 1 1 1
  spline S152 degree 3 poles (76.2227, -29.1679) (77.824, -29.3838) (80.1399, -30.7346) (86.8042, -30.7346) knots 0 0 0 0 1 1 1 1
  line L174 (98.4165, -35.8063) -> (98.4165, -33.2374)
  line L175 (98.4165, -33.2374) -> (-93.2285, -33.2375)
  line L176 (-93.2285, -33.2375) -> (-93.2285, -35.8063)
  line L177 (-93.2285, -35.8063) -> (98.4165, -35.8063)
extrude "Extrude3" [suppressed] in component "Front"
extrude "Extrude26" [suppressed]
copy_body "CutPasteBodies2" [suppressed] in component "Front"
component "Front" placed x (1, 0, 0) y (0, 1, 0) z (0, 0, 1) at (0, 0, 0)
component "back" placed x (1, 0, 0) y (0, 1, 0) z (0, 0, 1) at (0, 0, 0)
component "feet" placed x (1, 0, 0) y (0, 1, 0) z (0, 0, 1) at (0, 0, 0)
